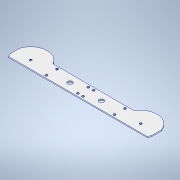
# Autodesk Inventor part: sidePanelv2
Saved by Autodesk Inventor 2020 (Build 240168000, 168)
## iProperties
Created: 2019-11-15
Part Number: sidePanelv2
Material: Aluminum 6061
Document SubType Name: Modeling
Designer: xj82b
Density: 2.7 g/cm^3
Appearance: Aluminum - Flat
Author: xj82b
Autodesk Inventor part; units mm, degrees
ref_plane "YZ Plane" through (0, 0, 0) normal (1, 0, 0) x (0, 1, 0)
ref_plane "XZ Plane" through (0, 0, 0) normal (0, 1, 0) x (-1, 0, 0)
ref_plane "XY Plane" through (0, 0, 0) normal (0, 0, 1) x (1, 0, 0)
sketch "Sketch1" plane through (0, 0, 0) normal (0, 1, 0) x (-1, 0, 0)
  line L0 (-4.1366, 0) -> (-427.8634, 0)
  line L1 (-432, -10) -> (-432, -38)
  line L2 (0, -38) -> (0, -10)
  circle A0 centre (-112, -40) radius 2
  circle A1 centre (-112, -8) radius 2
  circle A2 centre (-208, -40) radius 2
  circle A3 centre (-224, -40) radius 2
  circle A4 centre (-224, -8) radius 2
  circle A5 centre (-208, -8) radius 2
  circle A6 centre (-320, -40) radius 2
  circle A7 centre (-320, -8) radius 2
  circle A8 centre (-48, -24) radius 2
  circle A9 centre (-384, -24) radius 2
  circle A10 centre (-168, -24) radius 7
  circle A11 centre (-264, -24) radius 7
  arc A12 (-91.8634, -48) -> (0, -38) centre (-48, -24) ccw
  arc A13 (0, -10) -> (-4.1366, 0) centre (-48, -24) ccw
  line L3 (-340.1366, -48) -> (-91.8634, -48)
  arc A14 (-427.8634, 0) -> (-432, -10) centre (-384, -24) ccw
  arc A15 (-432, -38) -> (-340.1366, -48) centre (-384, -24) ccw
  point P0 (0, 0)
  point P1 (0, 0)
  point P2 (-432, -48)
  point P3 (-432, 0)
  point P4 (0, -48)
  point P5 (0, -24)
  point P6 (-432, -24)
  dimension "d0" = 432
  dimension "d1" = 48
  dimension "d2" = 4
  dimension "d3" = 4
  dimension "d4" = 4
  dimension "d5" = 4
  dimension "d6" = 4
  dimension "d7" = 4
  dimension "d8" = 4
  dimension "d9" = 4
  dimension "d10" = 208
  dimension "d11" = 208
  dimension "d14" = 8
  dimension "d15" = 112
  dimension "d16" = 112
  dimension "d17" = 4
  dimension "d18" = 48
  dimension "d19" = 4
  dimension "d20" = 48
  dimension "d21" = 14
  dimension "d22" = 14
  dimension "d23" = 168
  dimension "d24" = 168
  constraints: 16 centre point, 9 horizontal alignment, 8 end point, 8 point on circle, 6 point on line, 4 vertical alignment, 2 midpoint, 2 parallel, 1 horizontal, 1 perpendicular
  measures "d0" distance of point (0, -48) point (-432, -48)
  measures "d1" distance of point (-432, -48) point (-432, 0)
  measures "d2" diameter of A0
  measures "d3" diameter of A1
  measures "d4" diameter of A2
  measures "d5" diameter of A3
  measures "d6" diameter of A4
  measures "d7" diameter of A5
  measures "d8" diameter of A6
  measures "d9" diameter of A7
  measures "d10" distance from line of L2 A2.centre
  measures "d11" distance from line of L1 A3.centre
  measures "d14" distance from line of L0 A4.centre
  measures "d15" distance from line of L2 A0.centre
  measures "d16" distance from line of L1 A6.centre
  measures "d17" diameter of A8
  measures "d18" distance from line of L2 A8.centre
  measures "d19" diameter of A9
  measures "d20" distance from line of L1 A9.centre
  measures "d21" diameter of A10
  measures "d22" diameter of A11
  measures "d23" distance from line of L1 A11.centre
  measures "d24" distance from line of L2 A10.centre
extrude "Extrusion1" add sketch "Sketch1" along normal blind 3.175
sketch "Sketch2" plane through (0, 3.175, 0) normal (0, 1, 0) x (1, 0, 0)
  circle A0 centre (47.9691, 23.9283) radius 3.5
  circle A1 centre (112, 8) radius 2 projected
  circle A2 centre (112, 8) radius 3.5
  circle A3 centre (112, 40) radius 2 projected
  circle A4 centre (112, 40) radius 3.5
  circle A5 centre (208, 40) radius 2 projected
  circle A6 centre (208, 40) radius 3.5
  circle A7 centre (224, 40) radius 2 projected
  circle A8 centre (224, 40) radius 3.5
  circle A9 centre (224, 8) radius 2 projected
  circle A10 centre (224, 8) radius 3.5
  circle A11 centre (208, 8) radius 2 projected
  circle A12 centre (208, 8) radius 3.5
  circle A13 centre (320, 40) radius 2 projected
  circle A14 centre (320, 40) radius 3.5
  circle A15 centre (320, 8) radius 2 projected
  circle A16 centre (320, 8) radius 3.5
  circle A17 centre (384, 24) radius 2 projected
  circle A18 centre (384, 24) radius 3.5
  point P0 (0, 0)
  dimension "d28" = 7
  dimension "d29" = 7
  dimension "d30" = 7
  dimension "d31" = 7
  dimension "d32" = 7
  dimension "d33" = 7
  dimension "d34" = 7
  dimension "d35" = 7
  dimension "d36" = 7
  dimension "d37" = 7
  constraints: 10 centre point, 9 coincident
  measures "d28" diameter of A0
  measures "d29" diameter of A2
  measures "d30" diameter of A4
  measures "d31" diameter of A6
  measures "d32" diameter of A8
  measures "d33" diameter of A10
  measures "d34" diameter of A12
  measures "d35" diameter of A14
  measures "d36" diameter of A16
  measures "d37" diameter of A18
extrude "Extrusion2" cut sketch "Sketch2" against normal blind 0.675
body "Solid1"
